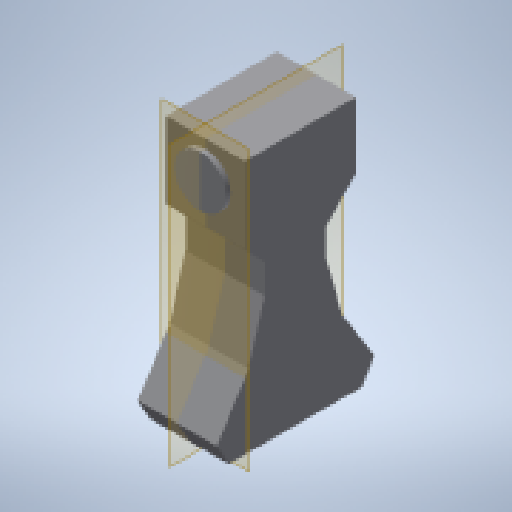
# Autodesk Inventor part: BaseBoundingBox
Saved by Autodesk Inventor 2023 (Build 270158000, 158)
## iProperties
Created: 2023-03-25
Part Number: BaseBoundingBox
Material: Generic
Document SubType Name: Modeling
Designer: Val
Density: 1 g/cm^3
Appearance: Default
Author: Val
Autodesk Inventor part; units mm, degrees
ref_plane "XZ Plane" through (0, 0, 0) normal (0, 1, 0) x (-1, 0, 0)
sketch "Sketch1" plane through (0, 0, 0) normal (1, 0, 0) x (0, 1, 0)
  line L0 (-16, 3.08) -> (16, 3.08)
  line L1 (16, 3.08) -> (16, 0)
  line L2 (16, 0) -> (-16, 0)
  line L3 (-16, 0) -> (-16, 3.08)
  line L4 (-20.328, 3.08) -> (15.75, 3.08) construction
  line L5 (16, 0) -> (-16, 0) construction
  line L6 (-16, 0) -> (-25.6061, 0)
  line L7 (-25.6061, 0) -> (-38.4616, -12.16)
  line L8 (-38.4616, -12.16) -> (-56.7976, -12.16)
  line L9 (-56.7976, -50.84) -> (-38.4616, -50.84)
  line L10 (-38.4616, -50.84) -> (-19.263, -69)
  line L11 (-19.263, -69) -> (21.5, -69)
  line L12 (21.5, -69) -> (21.5, 0)
  line L13 (21.5, 0) -> (16, 0)
  line L14 (-19.5, -69) -> (19.5, -69) construction
  line L15 (-36.9927, -10.7705) -> (-23.8189, 1.6905) construction
  line L16 (-23.8189, -64.6905) -> (-36.9927, -52.2295) construction
  line L17 (-56.7976, -12.16) -> (-40.4836, -12.16) construction
  line L18 (-40.4836, -50.84) -> (-56.7976, -50.84) construction
  line L19 (-133.6344, 11.4742) -> (-125.5921, 15.9321) construction
  line L20 (-125.5921, -78.9321) -> (-133.6344, -74.4742) construction
  line L21 (-56.7976, -12.16) -> (-91.2748, -2.4786)
  line L22 (-91.2748, -2.4786) -> (-122.9717, 17.3846)
  line L23 (-122.9717, 17.3846) -> (-136.2516, 10.0235)
  line L24 (-136.2516, 10.0235) -> (-136.2516, -73.0235)
  line L25 (-136.2516, -73.0235) -> (-122.9717, -80.3846)
  line L26 (-122.9717, -80.3846) -> (-91.2748, -60.5214)
  line L27 (-91.2748, -60.5214) -> (-56.7976, -50.84)
  line L28 (-91.2748, -2.4786) -> (-58.1979, -11.9632) construction
  line L29 (-120.3625, 15.7495) -> (-94.6911, -0.9217) construction
  line L30 (-136.2516, -70.0311) -> (-136.2516, 7.0311) construction
  line L31 (-94.6911, -62.0783) -> (-120.3625, -78.7495) construction
  line L32 (-58.1979, -51.0368) -> (-91.2748, -60.5214) construction
  point P0 (0, 0)
  point P1 (0, 0)
  point P2 (21.5, -10)
  point P3 (-129.6132, 13.7032)
  point P4 (-129.6132, -76.7032)
  point P5 (16, 0)
  point P6 (16, 0)
  constraints: 38 end point, 9 collinear, 5 parallel, 4 point on line, 3 midpoint, 3 perpendicular, 2 horizontal, 1 coincident, 1 vertical, 1 other
extrude "Extrusion3" add sketch "Sketch1" along normal mid plane 49 contours L2 L13 L12 L11 L10 L9 L27 L26 L25 L24 L23 L22 L21 L8 L7 L6
sketch "Sketch3" plane through (-24.5, -25.6061, 0) normal (0, 0, 1) x (1, 0, 0)
  circle A0 centre (24.5, 25.6061) radius 16 projected
extrude "Extrusion4" add sketch "Sketch3" along normal up to surface (3.08 mm away)
body "Solid2"
